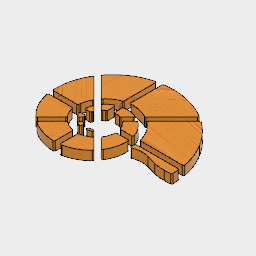
logo (Autodesk Fusion 360 design; units mm, degrees)
Autodesk Fusion 360 part; units mm, degrees
note: some values were not read from the file. Set by a fixed rule: which sketch regions a step uses.
sketch "草图1" plane through (0, 0, 0) normal (0, 1, 0) x (1, 0, 0)
  spline S0 degree 3 poles (12.3773, -27.2777) (11.6975, -26.3895) (11.2331, -25.3673) (10.9888, -24.277) knots 0 0 0 0 1 1 1 1
  spline S1 degree 3 poles (10.9888, -24.277) (10.9504, -24.1053) (10.8021, -23.9811) (10.6262, -23.9811) knots 0 0 0 0 1 1 1 1
  line L0 (10.6262, -23.9811) -> (3.069, -23.9811)
  spline S2 degree 3 poles (3.069, -23.9811) (2.8342, -23.9811) (2.6606, -24.1963) (2.7053, -24.427) knots 0 0 0 0 1 1 1 1
  spline S3 degree 3 poles (2.7053, -24.427) (3.2911, -27.4595) (4.9062, -30.3545) (7.1472, -32.4709) knots 0 0 0 0 1 1 1 1
  spline S4 degree 3 poles (7.1472, -32.4709) (7.2922, -32.6078) (7.521, -32.6013) (7.6618, -32.4605) knots 0 0 0 0 1 1 1 1
  line L1 (7.6618, -32.4605) -> (12.3503, -27.7718)
  spline S5 degree 3 poles (12.3503, -27.7718) (12.4839, -27.6381) (12.4922, -27.4277) (12.3773, -27.2777) knots 0 0 0 0 1 1 1 1
  line L2 (12.3773, -27.2777) -> (12.3773, -27.2777)
  spline S6 degree 3 poles (10.4926, -22.2705) (10.6875, -22.2705) (10.8486, -22.1193) (10.8614, -21.9246) knots 0 0 0 0 1 1 1 1
  spline S7 degree 3 poles (10.8614, -21.9246) (10.8733, -21.7457) (10.8858, -21.5671) (10.8992, -21.3882) knots 0 0 0 0 1 1 1 1
  line L3 (10.8992, -21.3882) -> (10.9245, -21.3892)
  spline S8 degree 3 poles (10.9245, -21.3892) (11.1665, -20.3584) (11.429, -19.3687) (11.9145, -18.4269) knots 0 0 0 0 1 1 1 1
  spline S9 degree 3 poles (11.9145, -18.4269) (11.9895, -18.2814) (11.9663, -18.1046) (11.8505, -17.9888) knots 0 0 0 0 1 1 1 1
  line L4 (11.8505, -17.9888) -> (5.5569, -11.6954)
  spline S10 degree 3 poles (5.5569, -11.6954) (5.3859, -11.5246) (5.0976, -11.5582) (4.9761, -11.7669) knots 0 0 0 0 1 1 1 1
  spline S11 degree 3 poles (4.9761, -11.7669) (3.1859, -14.8422) (2.3086, -18.3659) (2.4208, -21.9137) knots 0 0 0 0 1 1 1 1
  spline S12 degree 3 poles (2.4208, -21.9137) (2.4273, -22.1131) (2.5933, -22.2706) (2.7928, -22.2706) knots 0 0 0 0 1 1 1 1
  line L5 (2.7928, -22.2706) -> (10.4926, -22.2706)
  line L6 (10.4926, -22.2706) -> (10.4926, -22.2705)
  spline S13 degree 3 poles (17.044, -30.2379) (15.965, -30.0063) (14.972, -29.5378) (14.065, -28.9106) knots 0 0 0 0 1 1 1 1
  spline S14 degree 3 poles (14.065, -28.9106) (13.9159, -28.8073) (13.7156, -28.8219) (13.5873, -28.9499) knots 0 0 0 0 1 1 1 1
  line L7 (13.5873, -28.9499) -> (9.0537, -33.4838)
  spline S15 degree 3 poles (9.0537, -33.4838) (8.8903, -33.6472) (8.9123, -33.9217) (9.1037, -34.0511) knots 0 0 0 0 1 1 1 1
  spline S16 degree 3 poles (9.1037, -34.0511) (11.4606, -35.6424) (14.1341, -36.4395) (16.9529, -36.6154) knots 0 0 0 0 1 1 1 1
  spline S17 degree 3 poles (16.9529, -36.6154) (17.1654, -36.6288) (17.3443, -36.4571) (17.3443, -36.2443) knots 0 0 0 0 1 1 1 1
  line L8 (17.3443, -36.2443) -> (17.3443, -30.6016)
  spline S18 degree 3 poles (17.3443, -30.6016) (17.3443, -30.4239) (17.2175, -30.2751) (17.044, -30.2379) knots 0 0 0 0 1 1 1 1
  spline S19 degree 3 poles (34.0491, -5.4208) (29.6968, -2.8585) (24.3991, -1.6373) (19.3764, -2.2915) knots 0 0 0 0 1 1 1 1
  spline S20 degree 3 poles (19.3764, -2.2915) (19.1922, -2.3153) (19.055, -2.4746) (19.055, -2.6606) knots 0 0 0 0 1 1 1 1
  line L9 (19.055, -2.6606) -> (19.055, -12.9714)
  spline S21 degree 3 poles (19.055, -12.9714) (19.055, -13.1833) (19.2321, -13.3551) (19.4434, -13.3417) knots 0 0 0 0 1 1 1 1
  spline S22 degree 3 poles (19.4434, -13.3417) (21.4118, -13.2155) (23.4213, -13.6873) (25.1807, -14.5767) knots 0 0 0 0 1 1 1 1
  spline S23 degree 3 poles (25.1807, -14.5767) (25.3248, -14.6493) (25.4983, -14.624) (25.6123, -14.51) knots 0 0 0 0 1 1 1 1
  line L10 (25.6123, -14.51) -> (34.1202, -6.0021)
  spline S24 degree 3 poles (34.1202, -6.0021) (34.2908, -5.8315) (34.2572, -5.5434) (34.0491, -5.4208) knots 0 0 0 0 1 1 1 1
  spline S25 degree 3 poles (19.7562, -36.4217) (22.228, -35.824) (24.4777, -34.7533) (26.2315, -32.8852) knots 0 0 0 0 1 1 1 1
  spline S26 degree 3 poles (26.2315, -32.8852) (26.3699, -32.7376) (26.3696, -32.5081) (26.2264, -32.3649) knots 0 0 0 0 1 1 1 1
  line L11 (26.2264, -32.3649) -> (22.9656, -29.1044)
  spline S27 degree 3 poles (22.9656, -29.1044) (22.8346, -28.9734) (22.625, -28.9567) (22.4795, -29.0716) knots 0 0 0 0 1 1 1 1
  spline S28 degree 3 poles (22.4795, -29.0716) (21.5728, -29.7878) (20.5036, -30.2066) (19.3663, -30.3727) knots 0 0 0 0 1 1 1 1
  spline S29 degree 3 poles (19.3663, -30.3727) (19.1862, -30.3989) (19.055, -30.5566) (19.055, -30.7385) knots 0 0 0 0 1 1 1 1
  line L12 (19.055, -30.7385) -> (19.055, -36.0928)
  spline S30 degree 3 poles (19.055, -36.0928) (19.055, -36.3166) (19.2514, -36.4892) (19.4735, -36.4607) knots 0 0 0 0 1 1 1 1
  line L13 (19.4735, -36.4607) -> (19.7125, -36.4297)
  spline S31 degree 3 poles (19.7125, -36.4297) (19.7271, -36.4278) (19.7416, -36.4252) (19.7562, -36.4217) knots 0 0 0 0 1 1 1 1
  line L14 (19.7562, -36.4217) -> (19.7562, -36.4217)
  spline S32 degree 3 poles (24.3125, -26.8529) (24.222, -27.0259) (24.1264, -27.1911) (24.0243, -27.3506) knots 0 0 0 0 1 1 1 1
  spline S33 degree 3 poles (24.0243, -27.3506) (23.9318, -27.4953) (23.9583, -27.6855) (24.0806, -27.8063) knots 0 0 0 0 1 1 1 1
  spline S34 degree 3 poles (24.0806, -27.8063) (25.128, -28.8404) (26.1648, -29.886) (27.2051, -30.9281) knots 0 0 0 0 1 1 1 1
  spline S35 degree 3 poles (27.2051, -30.9281) (27.3765, -31.0999) (27.6638, -31.063) (27.7885, -30.8546) knots 0 0 0 0 1 1 1 1
  spline S36 degree 3 poles (27.7885, -30.8546) (28.9488, -28.9175) (29.606, -26.5856) (29.4479, -24.3202) knots 0 0 0 0 1 1 1 1
  spline S37 degree 3 poles (29.4479, -24.3202) (29.4342, -24.1282) (29.2699, -23.9811) (29.0773, -23.9811) knots 0 0 0 0 1 1 1 1
  line L15 (29.0773, -23.9811) -> (25.3927, -23.9811)
  spline S38 degree 3 poles (25.3927, -23.9811) (25.1956, -23.9811) (25.0349, -24.135) (25.023, -24.3318) knots 0 0 0 0 1 1 1 1
  spline S39 degree 3 poles (25.023, -24.3318) (25.0128, -24.4988) (24.9968, -24.6657) (24.9858, -24.8318) knots 0 0 0 0 1 1 1 1
  line L16 (24.9858, -24.8318) -> (24.9643, -24.8311)
  spline S40 degree 3 poles (24.9643, -24.8311) (24.8721, -25.4651) (24.6964, -26.3379) (24.3125, -26.8528) knots 0 0 0 0 1 1 1 1
  spline S41 degree 3 poles (24.3125, -26.8528) (24.1755, -27.1144) (24.3473, -26.8061) (24.3125, -26.8528) knots 0 0 0 0 1 1 1 1
  line L17 (24.3125, -26.8528) -> (24.3125, -26.8529)
  spline S42 degree 3 poles (13.2748, -16.4492) (14.313, -15.2845) (15.626, -14.3787) (17.0952, -13.8477) knots 0 0 0 0 1 1 1 1
  spline S43 degree 3 poles (17.0952, -13.8477) (17.2434, -13.7941) (17.3443, -13.656) (17.3443, -13.4986) knots 0 0 0 0 1 1 1 1
  line L18 (17.3443, -13.4986) -> (17.3443, -3.1345)
  spline S44 degree 3 poles (17.3443, -3.1345) (17.3443, -2.8943) (17.1184, -2.7142) (16.8856, -2.7737) knots 0 0 0 0 1 1 1 1
  spline S45 degree 3 poles (16.8856, -2.7737) (12.7539, -3.8319) (9.0159, -6.2965) (6.3941, -9.6597) knots 0 0 0 0 1 1 1 1
  spline S46 degree 3 poles (6.3941, -9.6597) (6.2792, -9.807) (6.2945, -10.0178) (6.4264, -10.1496) knots 0 0 0 0 1 1 1 1
  line L19 (6.4264, -10.1496) -> (12.739, -16.462)
  spline S47 degree 3 poles (12.739, -16.462) (12.8884, -16.6118) (13.134, -16.6073) (13.2748, -16.4492) knots 0 0 0 0 1 1 1 1
  line L20 (13.2748, -16.4492) -> (13.2748, -16.4492)
  spline S48 degree 3 poles (28.9589, -21.7779) (28.3478, -19.9931) (27.206, -18.4161) (25.6876, -17.2898) knots 0 0 0 0 1 1 1 1
  spline S49 degree 3 poles (25.6876, -17.2898) (25.5418, -17.1815) (25.337, -17.2005) (25.2084, -17.3291) knots 0 0 0 0 1 1 1 1
  line L21 (25.2084, -17.3291) -> (23.1635, -19.374)
  spline S50 degree 3 poles (23.1635, -19.374) (23.012, -19.5255) (23.0206, -19.7723) (23.1817, -19.9137) knots 0 0 0 0 1 1 1 1
  spline S51 degree 3 poles (23.1817, -19.9137) (23.8368, -20.4872) (24.3533, -21.221) (24.6679, -22.0261) knots 0 0 0 0 1 1 1 1
  spline S52 degree 3 poles (24.6679, -22.0261) (24.7247, -22.1717) (24.8602, -22.2705) (25.0161, -22.2705) knots 0 0 0 0 1 1 1 1
  line L22 (25.0161, -22.2705) -> (28.6068, -22.2705)
  spline S53 degree 3 poles (28.6068, -22.2705) (28.8616, -22.2705) (29.0413, -22.019) (28.9589, -21.7779) knots 0 0 0 0 1 1 1 1
  line L23 (28.9589, -21.7779) -> (28.9589, -21.7779)
  spline S54 degree 3 poles (23.4746, -16.6478) (23.6657, -16.4567) (23.5963, -16.1281) (23.3418, -16.037) knots 0 0 0 0 1 1 1 1
  spline S55 degree 3 poles (23.3418, -16.037) (22.361, -15.686) (21.3326, -15.5146) (20.287, -15.5009) knots 0 0 0 0 1 1 1 1
  line L24 (20.287, -15.5009) -> (20.287, -15.4973)
  spline S56 degree 3 poles (20.287, -15.4973) (19.9872, -15.5259) (19.6887, -15.5402) (19.3901, -15.57) knots 0 0 0 0 1 1 1 1
  spline S57 degree 3 poles (19.3901, -15.57) (19.1999, -15.5887) (19.055, -15.7488) (19.055, -15.9399) knots 0 0 0 0 1 1 1 1
  line L25 (19.055, -15.9399) -> (19.055, -18.1572)
  spline S58 degree 3 poles (19.055, -18.1572) (19.055, -18.3652) (19.2264, -18.5313) (19.4345, -18.5266) knots 0 0 0 0 1 1 1 1
  spline S59 degree 3 poles (19.4345, -18.5266) (19.9956, -18.5135) (20.5412, -18.5822) (21.0817, -18.7501) knots 0 0 0 0 1 1 1 1
  spline S60 degree 3 poles (21.0817, -18.7501) (21.2159, -18.7918) (21.3618, -18.7602) (21.4612, -18.6611) knots 0 0 0 0 1 1 1 1
  line L26 (21.4612, -18.6611) -> (23.4746, -16.6478)
  spline S61 degree 3 poles (15.1369, -22.0011) (15.1673, -21.8907) (15.2021, -21.7803) (15.2414, -21.6701) knots 0 0 0 0 1 1 1 1
  spline S62 degree 3 poles (15.2414, -21.6701) (15.2887, -21.5377) (15.2515, -21.3897) (15.1521, -21.2903) knots 0 0 0 0 1 1 1 1
  line L27 (15.1521, -21.2903) -> (14.0752, -20.2134)
  spline S63 degree 3 poles (14.0752, -20.2134) (13.8787, -20.0172) (13.5483, -20.0994) (13.459, -20.3622) knots 0 0 0 0 1 1 1 1
  spline S64 degree 3 poles (13.459, -20.3622) (13.2944, -20.8465) (13.1852, -21.3522) (13.1349, -21.8624) knots 0 0 0 0 1 1 1 1
  spline S65 degree 3 poles (13.1349, -21.8624) (13.1134, -22.0809) (13.2858, -22.2705) (13.5055, -22.2705) knots 0 0 0 0 1 1 1 1
  line L28 (13.5055, -22.2705) -> (14.7812, -22.2705)
  spline S66 degree 3 poles (14.7812, -22.2705) (14.947, -22.2705) (15.0929, -22.161) (15.1369, -22.0011) knots 0 0 0 0 1 1 1 1
  spline S67 degree 3 poles (15.2447, -24.5556) (15.2027, -24.4538) (15.1643, -24.3496) (15.1316, -24.2446) knots 0 0 0 0 1 1 1 1
  spline S68 degree 3 poles (15.1316, -24.2446) (15.083, -24.0883) (14.9411, -23.9811) (14.7776, -23.9811) knots 0 0 0 0 1 1 1 1
  line L29 (14.7776, -23.9811) -> (13.7879, -23.9811)
  spline S69 degree 3 poles (13.7879, -23.9811) (13.534, -23.9811) (13.3504, -24.2315) (13.4358, -24.4705) knots 0 0 0 0 1 1 1 1
  spline S70 degree 3 poles (13.4358, -24.4705) (13.5689, -24.8431) (13.7394, -25.2015) (13.951, -25.5361) knots 0 0 0 0 1 1 1 1
  spline S71 degree 3 poles (13.951, -25.5361) (14.0773, -25.7358) (14.3591, -25.7632) (14.5261, -25.5962) knots 0 0 0 0 1 1 1 1
  line L30 (14.5261, -25.5962) -> (15.1643, -24.958)
  spline S72 degree 3 poles (15.1643, -24.958) (15.27, -24.8521) (15.3015, -24.6937) (15.2447, -24.5556) knots 0 0 0 0 1 1 1 1
  spline S73 degree 3 poles (17.1422, -26.6374) (16.969, -26.5478) (16.8026, -26.4451) (16.6445, -26.3311) knots 0 0 0 0 1 1 1 1
  spline S74 degree 3 poles (16.6445, -26.3311) (16.4978, -26.2252) (16.296, -26.2415) (16.1677, -26.3698) knots 0 0 0 0 1 1 1 1
  line L31 (16.1677, -26.3698) -> (15.7679, -26.7696)
  spline S75 degree 3 poles (15.7679, -26.7696) (15.5959, -26.9413) (15.6337, -27.2286) (15.8426, -27.3527) knots 0 0 0 0 1 1 1 1
  spline S76 degree 3 poles (15.8426, -27.3527) (16.1617, -27.5426) (16.5049, -27.703) (16.8583, -27.8161) knots 0 0 0 0 1 1 1 1
  spline S77 degree 3 poles (16.8583, -27.8161) (17.0985, -27.8929) (17.3443, -27.7143) (17.3443, -27.4622) knots 0 0 0 0 1 1 1 1
  line L32 (17.3443, -27.4622) -> (17.3443, -26.9592)
  spline S78 degree 3 poles (17.3443, -26.9592) (17.3443, -26.822) (17.264, -26.7005) (17.1422, -26.6374) knots 0 0 0 0 1 1 1 1
  spline S79 degree 3 poles (19.508, -27.9379) (19.9185, -27.8352) (20.3126, -27.673) (20.6736, -27.4518) knots 0 0 0 0 1 1 1 1
  spline S80 degree 3 poles (20.6736, -27.4518) (20.8748, -27.3286) (20.9019, -27.0455) (20.7358, -26.8779) knots 0 0 0 0 1 1 1 1
  spline S81 degree 3 poles (20.7358, -26.8779) (20.6275, -26.7687) (20.4626, -26.7371) (20.3227, -26.8011) knots 0 0 0 0 1 1 1 1
  spline S82 degree 3 poles (20.3227, -26.8011) (20.0268, -26.9366) (19.711, -27.0258) (19.3842, -27.0666) knots 0 0 0 0 1 1 1 1
  spline S83 degree 3 poles (19.3842, -27.0666) (19.1969, -27.0898) (19.055, -27.2452) (19.055, -27.4339) knots 0 0 0 0 1 1 1 1
  line L33 (19.055, -27.4339) -> (19.055, -27.5756)
  spline S84 degree 3 poles (19.055, -27.5756) (19.055, -27.8134) (19.277, -27.9956) (19.508, -27.9379) knots 0 0 0 0 1 1 1 1
  spline S85 degree 3 poles (15.9968, -19.7202) (16.1382, -19.8613) (16.3639, -19.8634) (16.5112, -19.7288) knots 0 0 0 0 1 1 1 1
  spline S86 degree 3 poles (16.5112, -19.7288) (16.6794, -19.5752) (16.8591, -19.4344) (17.0482, -19.3073) knots 0 0 0 0 1 1 1 1
  spline S87 degree 3 poles (17.0482, -19.3073) (17.2056, -19.2011) (17.2964, -19.1924) (17.3443, -19.0439) knots 0 0 0 0 1 1 1 1
  spline S88 degree 2 poles (17.3443, -19.0439) (17.4295, -18.7793) (17.3443, -16.7305) knots 0 0 0 1 1 1
  spline S89 degree 3 poles (17.3443, -16.7305) (17.3443, -16.4457) (17.0383, -16.2706) (16.7886, -16.4081) knots 0 0 0 0 1 1 1 1
  spline S90 degree 3 poles (16.7886, -16.4081) (16.0355, -16.8231) (15.3563, -17.3734) (14.794, -18.0238) knots 0 0 0 0 1 1 1 1
  spline S91 degree 3 poles (14.794, -18.0238) (14.6654, -18.1724) (14.6708, -18.3941) (14.8098, -18.5331) knots 0 0 0 0 1 1 1 1
  line L34 (14.8098, -18.5331) -> (15.9968, -19.7202)
  line L35 (15.9968, -19.7202) -> (15.9968, -19.7202)
  spline S92 degree 3 poles (45.3517, -22.2705) (45.5794, -22.2705) (45.7565, -22.0669) (45.7184, -21.8422) knots 0 0 0 0 1 1 1 1
  spline S93 degree 3 poles (45.7184, -21.8422) (45.2347, -18.9882) (43.9804, -16.1462) (42.4769, -13.709) knots 0 0 0 0 1 1 1 1
  spline S94 degree 3 poles (42.4769, -13.709) (40.8342, -11.0465) (38.6806, -8.6825) (36.1678, -6.8162) knots 0 0 0 0 1 1 1 1
  spline S95 degree 3 poles (36.1678, -6.8162) (36.0205, -6.7067) (35.8139, -6.7233) (35.6841, -6.8534) knots 0 0 0 0 1 1 1 1
  line L36 (35.6841, -6.8534) -> (27.2101, -15.3274)
  spline S96 degree 3 poles (27.2101, -15.3274) (27.0533, -15.4842) (27.0676, -15.7435) (27.2426, -15.8798) knots 0 0 0 0 1 1 1 1
  spline S97 degree 3 poles (27.2426, -15.8798) (29.1878, -17.3949) (30.5981, -19.6044) (31.2065, -21.9883) knots 0 0 0 0 1 1 1 1
  spline S98 degree 3 poles (31.2065, -21.9883) (31.2487, -22.1535) (31.3946, -22.2705) (31.5652, -22.2705) knots 0 0 0 0 1 1 1 1
  line L37 (31.5652, -22.2705) -> (45.3517, -22.2705)
  spline S99 degree 3 poles (40.3148, -26.3597) (39.2369, -26.1308) (38.2258, -25.6977) (37.1569, -25.4438) knots 0 0 0 0 1 1 1 1
  spline S100 degree 3 poles (37.1569, -25.4438) (35.4671, -25.0426) (33.6312, -25.0706) (32.0155, -25.7358) knots 0 0 0 0 1 1 1 1
  spline S101 degree 3 poles (32.0155, -25.7358) (31.7676, -25.8379) (31.4985, -25.6424) (31.5107, -25.3748) knots 0 0 0 0 1 1 1 1
  spline S102 degree 3 poles (31.5107, -25.3748) (31.5253, -25.0518) (31.5342, -24.7024) (31.5294, -24.3589) knots 0 0 0 0 1 1 1 1
  spline S103 degree 3 poles (31.5294, -24.3589) (31.5265, -24.1514) (31.6922, -23.9811) (31.9, -23.9811) knots 0 0 0 0 1 1 1 1
  line L38 (31.9, -23.9811) -> (45.6711, -23.9811)
  spline S104 degree 3 poles (45.6711, -23.9811) (45.8601, -23.9811) (46.0211, -24.1231) (46.0414, -24.3109) knots 0 0 0 0 1 1 1 1
  spline S105 degree 3 poles (46.0414, -24.3109) (46.1086, -24.9396) (46.1464, -25.5685) (46.1833, -26.1996) knots 0 0 0 0 1 1 1 1
  spline S106 degree 3 poles (46.1833, -26.1996) (46.1949, -26.3954) (46.0521, -26.5657) (45.8574, -26.5898) knots 0 0 0 0 1 1 1 1
  spline S107 degree 3 poles (45.8574, -26.5898) (45.3731, -26.6499) (44.6567, -26.7136) (43.7935, -26.7136) knots 0 0 0 0 1 1 1 1
  spline S108 degree 3 poles (43.7935, -26.7136) (42.6257, -26.7136) (41.4572, -26.602) (40.3147, -26.3597) knots 0 0 0 0 1 1 1 1
extrude "拉伸1" add sketch "草图1" along normal blind 3 makes body 1 at (16.0954, 2.6667, 27.4941) makes body 2 at (22.4274, 0, 17.018) makes body 3 at (11.1722, 0, 32.5022) makes body 4 at (30.2677, 0, 8.1499) makes body 5 at (16.3092, 0, 6.7658) makes body 6 at (13.1538, 1.3333, 21.6925) makes body 7 at (27.3482, 0, 21.686) makes body 8 at (36.4904, 2, 23.9811) makes body 9 at (20.5521, 1.3333, 27.5233) makes body 10 at (16.5404, 1.3333, 16.5514) makes body 11 at (5.6428, 0, 24.7842) makes body 12 at (34.413, 0, 11.1005) makes body 13 at (7.0804, 0, 14.5888) makes body 14 at (13.5469, 2.6667, 24.7573) makes body 15 at (26.6088, 0, 29.3712) makes body 16 at (20.0078, 0, 34.1928)
